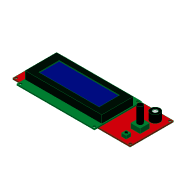
# Autodesk Inventor part: 2004A LCD Module
Saved by Autodesk Inventor 2015 (Build 190159000, 159)
## iProperties
Created: 2020-01-07
Part Number: 2004A LCD Module
Material: Generic
Document SubType Name: Modeling
Designer: Ghassan Yusuf
Density: 1 g/cm^3
Appearance: Default(1)
Author: Ghassan Yusuf
Autodesk Inventor part; units mm, degrees
ref_plane "YZ Plane" through (0, 0, 0) normal (1, 0, 0) x (0, 1, 0)
ref_plane "XZ Plane" through (0, 0, 0) normal (0, 1, 0) x (-1, 0, 0)
sketch "LCD Screen" plane through (0, 0, 0) normal (0, 0, 1) x (1, 0, 0)
  line L0 (-74.575, 27.52) -> (74.375, 27.52)
  line L1 (74.375, 27.52) -> (74.375, -27.6)
  line L2 (74.375, -27.6) -> (-74.575, -27.6)
  line L3 (-74.575, -27.6) -> (-74.575, 27.52)
  circle A0 centre (-72.5, 25.11) radius 1.6
  circle A1 centre (72.3, 25.11) radius 1.6
  circle A2 centre (72.3, -25.19) radius 1.6
  circle A3 centre (-72.5, -25.19) radius 1.6
  circle A4 centre (61.775, 16.9) radius 6.025
  line L4 (55.825, 3.7) -> (67.725, 3.7)
  line L5 (67.725, 3.7) -> (67.725, -8.2)
  line L6 (67.725, -8.2) -> (55.825, -8.2)
  line L7 (55.825, -8.2) -> (55.825, 3.7)
  line L8 (58.775, -17) -> (64.775, -17)
  line L9 (64.775, -17) -> (64.775, -23)
  line L10 (64.775, -23) -> (58.775, -23)
  line L11 (58.775, -23) -> (58.775, -17)
  line L12 (-61.575, 24.52) -> (36.975, 24.52)
  line L13 (36.975, 24.52) -> (36.975, -35.48)
  line L14 (36.975, -35.48) -> (-61.575, -35.48)
  line L15 (-61.575, -35.48) -> (-61.575, 24.52)
  line L16 (-60.9, 14.52) -> (36.3, 14.52)
  line L17 (36.3, 14.52) -> (36.3, -25.48)
  line L18 (36.3, -25.48) -> (-60.9, -25.48)
  line L19 (-60.9, -25.48) -> (-60.9, 14.52)
  line L20 (-50.55, 7.52) -> (25.95, 7.52)
  line L21 (25.95, 7.52) -> (25.95, -18.48)
  line L22 (25.95, -18.48) -> (-50.55, -18.48)
  line L23 (-50.55, -18.48) -> (-50.55, 7.52)
  line L24 (-74.575, -0.04) -> (74.375, -0.04)
  line L25 (-0.1, 27.52) -> (-0.1, -27.6)
  line L26 (55.825, -2.25) -> (67.725, -2.25)
  line L27 (61.775, 3.7) -> (61.775, -8.2)
  line L28 (61.775, -17) -> (61.775, -23)
  line L29 (58.775, -20) -> (64.775, -20)
  line L30 (-12.3, 24.52) -> (-12.3, -35.48)
  line L31 (-61.575, -5.48) -> (36.975, -5.48)
  point P0 (14.168, -4.3108)
  point P1 (-12.3, 7.52)
  point P2 (-12.3, 14.52)
  point P3 (-50.55, -5.48)
  point P4 (-60.9, -5.48)
  point P5 (61.775, -2.25)
  point P6 (61.775, -2.25)
  point P7 (61.775, -20)
  dimension "d0" = 148.95
  dimension "d1" = 55.12
  dimension "d2" = 3.2
  dimension "d3" = 3.2
  dimension "d4" = 3.2
  dimension "d5" = 3.2
  dimension "d11" = 12.05
  dimension "d14" = 11.9
  dimension "d15" = 11.9
  dimension "d17" = 6
  dimension "d18" = 6
  dimension "d21" = 60
  dimension "d23" = 13
  dimension "d24" = 97.2
  dimension "d25" = 40
  dimension "d27" = 26
  dimension "d28" = 76.5
  dimension "d59" = 50.3
  dimension "d60" = 25.15
  dimension "d61" = 144.8
  dimension "d62" = 72.4
  dimension "d63" = 13.2
  dimension "d64" = 8.8
  dimension "d65" = 9.6
  dimension "d66" = 3
  dimension "d67" = 10
  dimension "d68" = 4.6
  measures "d0" distance of L1.end L2.end
  measures "d1" distance of L0.end L1.end
  measures "d2" diameter of A0
  measures "d3" diameter of A1
  measures "d4" diameter of A2
  measures "d5" diameter of A3
  measures "d11" diameter of A4
  measures "d14" distance of L5.end L6.end
  measures "d15" distance of L4.end L5.end
  measures "d17" distance of L9.end L10.end
  measures "d18" distance of L8.end L9.end
  measures "d21" distance of L12.end L13.end
  measures "d23" distance between parallel lines of L3 L15
  measures "d24" distance of L17.end L18.end
  measures "d25" distance of L16.end L17.end
  measures "d27" distance of L20.end L21.end
  measures "d28" distance of L20.start L20.end
  measures "d59" distance of A3.centre A0.centre
  measures "d60" distance from line of L24 A0.centre
  measures "d61" distance of A1.centre A0.centre
  measures "d62" distance from line of L25 A0.centre
  measures "d63" distance from line of L4 A4.centre
  measures "d64" distance between parallel lines of L8 L6
  measures "d65" distance between parallel lines of L1 L9
  measures "d66" distance between parallel lines of L0 L12
  measures "d67" distance between parallel lines of L14 L18
  measures "d68" distance between parallel lines of L2 L10
sketch "Sketch1" plane through (0, 0, 0) normal (0, 0, 1) x (1, 0, 0)
  line L0 (-74.475, 27.48) -> (74.475, 27.56)
  line L1 (74.475, 27.56) -> (74.5046, -27.56)
  line L2 (74.5046, -27.56) -> (-74.4454, -27.64)
  line L3 (-74.4454, -27.64) -> (-74.475, 27.48)
  circle A0 centre (-72.3987, 25.0711) radius 1.6
  circle A1 centre (72.4013, 25.1489) radius 1.6
  circle A2 centre (72.4283, -25.1511) radius 1.6
  circle A3 centre (-72.3717, -25.2289) radius 1.6
  circle A4 centre (61.8807, 16.9332) radius 6.025
  line L4 (55.9378, 3.73) -> (67.8378, 3.7364)
  line L5 (67.8378, 3.7364) -> (67.8442, -8.1636)
  line L6 (67.8442, -8.1636) -> (55.9442, -8.17)
  line L7 (55.9442, -8.17) -> (55.9378, 3.73)
  line L8 (58.8989, -16.9684) -> (64.8989, -16.9652)
  line L9 (64.8989, -16.9652) -> (64.9021, -22.9652)
  line L10 (64.9021, -22.9652) -> (58.9021, -22.9684)
  line L11 (58.9021, -22.9684) -> (58.8989, -16.9684)
  line L12 (-61.4734, 24.487) -> (37.0766, 24.5399)
  line L13 (37.0766, 24.5399) -> (37.1088, -35.4601)
  line L14 (37.1088, -35.4601) -> (-61.4412, -35.513)
  line L15 (-61.4412, -35.513) -> (-61.4734, 24.487)
  line L16 (-60.793, 14.4873) -> (36.407, 14.5396)
  line L17 (36.407, 14.5396) -> (36.4285, -25.4604)
  line L18 (36.4285, -25.4604) -> (-60.7715, -25.5126)
  line L19 (-60.7715, -25.5126) -> (-60.793, 14.4873)
  line L20 (-50.4393, 7.4929) -> (26.0607, 7.534)
  line L21 (26.0607, 7.534) -> (26.0747, -18.466)
  line L22 (26.0747, -18.466) -> (-50.4253, -18.5071)
  line L23 (-50.4253, -18.5071) -> (-50.4393, 7.4929)
  line L24 (-74.4602, -0.08) -> (74.4898, 0)
  line L25 (0, 27.52) -> (0.0296, -27.6)
  line L26 (55.941, -2.22) -> (67.841, -2.2136)
  line L27 (61.8878, 3.7332) -> (61.8942, -8.1668)
  line L28 (61.8989, -16.9668) -> (61.9021, -22.9668)
  line L29 (58.9005, -19.9684) -> (64.9005, -19.9652)
  line L30 (-12.1984, 24.5134) -> (-12.1662, -35.4865)
  line L31 (-61.4573, -5.513) -> (37.0927, -5.4601)
  point P0 (0, 0)
  constraints: 2 other
extrude "Extrusion1" add sketch "Sketch1" against normal blind 1.6 contours L0 L25 L12 L15 L24 L3 | L0 L1 L24 L5 L4 L7 L13 L12 L25 | L24 L15 L2 L3 | L25 L16 L30 L12 | L12 L13 L24 L17 L16 L25 | L24 L19 L31 L15 | L15 L12 L30 L16 L19 L24 | L1 L2 L13 L24 L7 L6 L5 | L25 L20 L30 L16 | L16 L17 L24 L21 L20 L25 | L15 L31 L19 L18 L30 L2 | L24 L23 L31 L19 | L19 L16 L30 L20 L23 L24 | L24 L27 L4 L5 | L5 L26 L27 L24 | L13 L31 L17 L24 | L25 L24 L30 L20 | L20 L21 L24 L25 | L30 L18 L25 L2 | L31 L23 L22 L30 L18 L19 | L24 L30 L31 L23 | L23 L20 L30 L24 | L2 L25 L18 L17 L31 L13 | L5 L6 L27 L26 | L27 L26 L7 L24 | L24 L7 L4 L27 | L17 L31 L21 L24 | L25 L31 L30 L24 | L24 L21 L31 L25 | L30 L22 L25 L18 | L31 L30 L22 L23 | L27 L6 L7 L26 | L17 L18 L25 L22 L21 L31 | L31 L21 L22 L25 | L25 L22 L30 L31 | A4 | L8 L28 L29 L11 | L8 L9 L29 L28 | L29 L28 L10 L11 | L29 L9 L10 L28
extrude "Extrusion2" add sketch "Sketch1" along normal blind 9.7 contours A4
ref_plane "Work Plane1" through (0, 0, 4) normal (0, 0, 1) x (1, 0, 0)
sketch "Sketch2" plane through (0, 0, 4) normal (0, 0, 1) x (1, 0, 0)
  line L0 (-74.4454, -27.64) -> (-74.475, 27.48) projected
  line L1 (-74.475, 27.48) -> (74.475, 27.56) projected
  line L2 (-74.475, 27.48) -> (74.475, 27.56)
  line L3 (74.475, 27.56) -> (74.5046, -27.56)
  line L4 (74.5046, -27.56) -> (-74.4454, -27.64)
  line L5 (-74.4454, -27.64) -> (-74.475, 27.48)
  circle A0 centre (-72.3987, 25.0711) radius 1.6
  circle A1 centre (72.4013, 25.1489) radius 1.6
  circle A2 centre (72.4283, -25.1511) radius 1.6
  circle A3 centre (-72.3717, -25.2289) radius 1.6
  circle A4 centre (61.8807, 16.9332) radius 6.025
  line L6 (55.9378, 3.73) -> (67.8378, 3.7364)
  line L7 (67.8378, 3.7364) -> (67.8442, -8.1636)
  line L8 (67.8442, -8.1636) -> (55.9442, -8.17)
  line L9 (55.9442, -8.17) -> (55.9378, 3.73)
  line L10 (58.8989, -16.9684) -> (64.8989, -16.9652)
  line L11 (64.8989, -16.9652) -> (64.9021, -22.9652)
  line L12 (64.9021, -22.9652) -> (58.9021, -22.9684)
  line L13 (58.9021, -22.9684) -> (58.8989, -16.9684)
  line L14 (-61.4734, 24.487) -> (37.0766, 24.5399)
  line L15 (37.0766, 24.5399) -> (37.1088, -35.4601)
  line L16 (37.1088, -35.4601) -> (-61.4412, -35.513)
  line L17 (-61.4412, -35.513) -> (-61.4734, 24.487)
  line L18 (-60.793, 14.4873) -> (36.407, 14.5396)
  line L19 (36.407, 14.5396) -> (36.4285, -25.4604)
  line L20 (36.4285, -25.4604) -> (-60.7715, -25.5126)
  line L21 (-60.7715, -25.5126) -> (-60.793, 14.4873)
  line L22 (-50.4393, 7.4929) -> (26.0607, 7.534)
  line L23 (26.0607, 7.534) -> (26.0747, -18.466)
  line L24 (26.0747, -18.466) -> (-50.4253, -18.5071)
  line L25 (-50.4253, -18.5071) -> (-50.4393, 7.4929)
  line L26 (-74.4602, -0.08) -> (74.4898, 0)
  line L27 (0, 27.52) -> (0.0296, -27.6)
  line L28 (55.941, -2.22) -> (67.841, -2.2136)
  line L29 (61.8878, 3.7332) -> (61.8942, -8.1668)
  line L30 (61.8989, -16.9668) -> (61.9021, -22.9668)
  line L31 (58.9005, -19.9684) -> (64.9005, -19.9652)
  line L32 (-12.1984, 24.5134) -> (-12.1662, -35.4865)
  line L33 (-61.4573, -5.513) -> (37.0927, -5.4601)
  point P0 (0, 0)
  constraints: 2 other
extrude "Extrusion3" add sketch "Sketch2" against normal blind 1.6 contours L17 L33 L21 L20 L32 L4 | L4 L32 L16 L17 | L26 L21 L33 L17 | L17 L14 L32 L18 L21 L26 | L32 L20 L27 L4 | L4 L15 L16 L32 | L26 L25 L33 L21 | L21 L18 L32 L22 L25 L26 | L27 L20 L19 L33 L15 L4 | L32 L24 L27 L20 | L20 L21 L33 L25 L24 L32 | L27 L18 L32 L14 | L14 L15 L26 L19 L18 L27 | L26 L32 L33 L25 | L25 L22 L32 L26 | L27 L24 L23 L33 L19 L20 | L32 L33 L27 L24 | L24 L25 L33 L32 | L27 L22 L32 L18 | L18 L19 L26 L23 L22 L27 | L32 L22 L27 L26 | L26 L27 L33 L32 | L33 L19 L26 L15 | L27 L33 L23 L24 | L22 L23 L26 L27 | L26 L23 L33 L27 | L33 L23 L26 L19
extrude "Extrusion4" add sketch "Sketch2" along normal blind 9.88 contours L26 L25 L33 L21 | L21 L18 L32 L22 L25 L26 | L32 L24 L27 L20 | L20 L21 L33 L25 L24 L32 | L26 L32 L33 L25 | L25 L22 L32 L26 | L27 L24 L23 L33 L19 L20 | L32 L33 L27 L24 | L24 L25 L33 L32 | L27 L22 L32 L18 | L18 L19 L26 L23 L22 L27 | L32 L22 L27 L26 | L26 L27 L33 L32 | L27 L33 L23 L24 | L22 L23 L26 L27 | L26 L23 L33 L27 | L33 L23 L26 L19
sketch "Sketch3" plane through (0, 0, 13.88) normal (0, 0, 1) x (1, 0, 0)
  line L0 (74.475, 27.56) -> (74.5046, -27.56) projected
  line L1 (-74.475, 27.48) -> (74.475, 27.56) projected
  line L2 (-74.4749, 27.32) -> (74.4749, 27.56)
  line L3 (74.4749, 27.56) -> (74.5637, -27.56)
  line L4 (74.5637, -27.56) -> (-74.3861, -27.7999)
  line L5 (-74.3861, -27.7999) -> (-74.4749, 27.32)
  circle A0 centre (-72.396, 24.9134) radius 1.6
  circle A1 centre (72.4038, 25.1466) radius 1.6
  circle A2 centre (72.4848, -25.1533) radius 1.6
  circle A3 centre (-72.315, -25.3866) radius 1.6
  circle A4 centre (61.892, 16.9197) radius 6.025
  line L6 (55.9633, 3.7101) -> (67.8633, 3.7293)
  line L7 (67.8633, 3.7293) -> (67.8824, -8.1707)
  line L8 (67.8824, -8.1707) -> (55.9825, -8.1899)
  line L9 (55.9825, -8.1899) -> (55.9633, 3.7101)
  line L10 (58.9466, -16.9851) -> (64.9466, -16.9754)
  line L11 (64.9466, -16.9754) -> (64.9563, -22.9754)
  line L12 (64.9563, -22.9754) -> (58.9563, -22.9851)
  line L13 (58.9563, -22.9851) -> (58.9466, -16.9851)
  line L14 (-61.4701, 24.341) -> (37.0798, 24.4997)
  line L15 (37.0798, 24.4997) -> (37.1764, -35.5002)
  line L16 (37.1764, -35.5002) -> (-61.3734, -35.6589)
  line L17 (-61.3734, -35.6589) -> (-61.4701, 24.341)
  line L18 (-60.779, 14.3421) -> (36.4209, 14.4986)
  line L19 (36.4209, 14.4986) -> (36.4853, -25.5013)
  line L20 (36.4853, -25.5013) -> (-60.7145, -25.6579)
  line L21 (-60.7145, -25.6579) -> (-60.779, 14.3421)
  line L22 (-50.4177, 7.3588) -> (26.0822, 7.482)
  line L23 (26.0822, 7.482) -> (26.1241, -18.518)
  line L24 (26.1241, -18.518) -> (-50.3758, -18.6412)
  line L25 (-50.3758, -18.6412) -> (-50.4177, 7.3588)
  line L26 (-74.4305, -0.2399) -> (74.5193, 0)
  line L27 (0, 27.44) -> (0.0888, -27.6799)
  line L28 (55.9729, -2.2399) -> (67.8729, -2.2207)
  line L29 (61.9133, 3.7197) -> (61.9325, -8.1803)
  line L30 (61.9466, -16.9803) -> (61.9563, -22.9803)
  line L31 (58.9515, -19.9851) -> (64.9515, -19.9754)
  line L32 (-12.1952, 24.4204) -> (-12.0985, -35.5796)
  line L33 (-61.4218, -5.659) -> (37.1281, -5.5002)
  point P0 (0, 0)
  point P1 (74.4898, 0)
  point P2 (0, 27.52)
  constraints: 2 midpoint, 2 other
extrude "Extrusion5" cut sketch "Sketch3" against normal blind 1 contours L27 L26 L32 L22 | L22 L23 L26 L27 | L32 L26 L25 L22 | L27 L33 L32 L26 | L26 L23 L33 L27 | L27 L33 L23 L24 | L24 L32 L33 L27 | L26 L32 L33 L25 | L24 L25 L33 L32
sketch "Sketch4" plane through (0, 0, 4) normal (0, 0, 1) x (1, 0, 0)
  circle A0 centre (-59.0221, 22.0383) radius 1.75
  circle A1 centre (34.6279, 22.0383) radius 1.75
  circle A2 centre (-59.0221, -33.0114) radius 1.75
  circle A3 centre (34.6279, -33.0114) radius 1.75
  line L0 (-61.4734, 24.487) -> (37.0766, 24.5399) projected
  line L1 (-61.4412, -35.513) -> (-61.4734, 24.487) projected
  line L2 (37.1088, -35.4601) -> (-61.4412, -35.513) projected
  line L3 (37.0766, 24.5399) -> (37.1088, -35.4601) projected
  point P0 (0, 0)
  dimension "d40" = 3.5
  dimension "d42" = 2.45
  dimension "d43" = 2.45
  dimension "d44" = 2.45
  dimension "d45" = 2.45
  constraints: 4 centre point, 3 equal radius, 2 horizontal alignment, 2 vertical alignment
  measures "d40" diameter of A0
  measures "d42" distance from line of A0.centre L0
  measures "d43" distance from line of L1 A0.centre
  measures "d44" distance from line of L2 A3.centre
  measures "d45" distance from line of L3 A1.centre
extrude "Extrusion6" cut sketch "Sketch4" against normal blind 2 contours A0 | A1 | A2 | A3
extrude "Extrusion7" add sketch "Sketch1" along normal blind 6 contours L24 L27 L4 L5 | L5 L26 L27 L24 | L5 L6 L27 L26 | L27 L26 L7 L24 | L24 L7 L4 L27 | L27 L6 L7 L26
extrude "Extrusion8" add sketch "Sketch1" along normal blind 4 contours L8 L28 L29 L11 | L8 L9 L29 L28 | L29 L28 L10 L11 | L29 L9 L10 L28
sketch "Sketch5" plane through (0, 0, 6) normal (0, 0, 1) x (1, 0, 0)
  circle A0 centre (61.8878, -2.2136) radius 3.4
  line L0 (67.8442, -8.1636) -> (67.8378, 3.7364) projected
  line L1 (67.8378, 3.7364) -> (55.9378, 3.73) projected
  point P0 (0, 0)
  point P1 (67.841, -2.2136)
  point P2 (61.8878, 3.7332)
  dimension "d52" = 6.8
  constraints: 2 midpoint, 1 centre point, 1 horizontal alignment, 1 vertical alignment
  measures "d52" diameter of A0
extrude "Extrusion9" add sketch "Sketch5" along normal blind 20
sketch "Sketch6" plane through (0, 0, 4) normal (0, 0, 1) x (1, 0, 0)
  circle A0 centre (61.8989, -19.9652) radius 1.75
  line L0 (64.8989, -16.9652) -> (58.8989, -16.9684) projected
  line L1 (64.9021, -22.9652) -> (64.8989, -16.9652) projected
  point P0 (0, 0)
  point P1 (61.8989, -16.9668)
  point P2 (64.9005, -19.9652)
  dimension "d55" = 3.5
  constraints: 2 midpoint, 1 centre point, 1 horizontal alignment, 1 vertical alignment
  measures "d55" diameter of A0
extrude "Extrusion10" add sketch "Sketch6" along normal blind 0.8
sketch "Sketch7" plane through (61.8807, 16.9332, 9.7) normal (0, 0, 1) x (1, 0, 0)
  circle A0 centre (0, 0) radius 3
  point P0 (-61.8807, -16.9332)
  dimension "d69" = 6
  constraints: 1 centre point
  measures "d69" diameter of A0
extrude "Extrusion11" cut sketch "Sketch7" against normal blind 1
equation "\"d60\" = 0.5 * d59"
equation "\"d62\" = 0.5 * d61"
equation "\"d43\" = d42"
equation "\"d44\" = d43"
equation "\"d45\" = d43"
body "Solid1"
